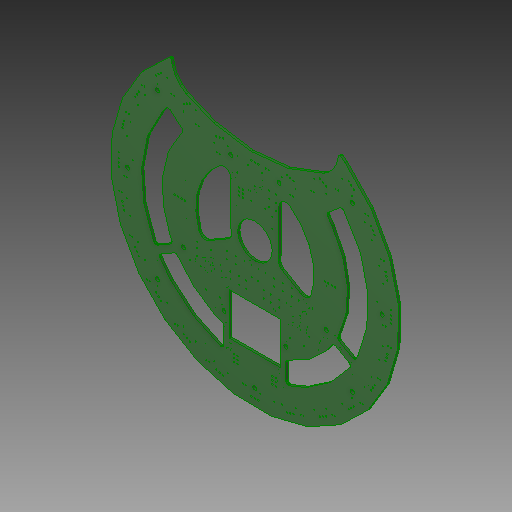
# Autodesk Inventor part: Board 2.brd_Outline
Saved by Autodesk Inventor 2017 (Build 210142000, 142)
## iProperties
Created: 2019-06-13
Part Number: Board 2.brd_Outline
Material: Generic
Document SubType Name: Modeling
Designer: Marc
Density: 1 g/cm^3
Appearance: Board Outline
Author: Marc
Autodesk Inventor part; units mm, degrees
ref_plane "YZ Plane" through (0, 0, 0) normal (1, 0, 0) x (0, 1, 0)
ref_plane "XZ Plane" through (0, 0, 0) normal (0, 1, 0) x (-1, 0, 0)
ref_plane "XY Plane" through (0, 0, 0) normal (0, 0, 1) x (1, 0, 0)
sketch "Sketch1" plane through (0, 0, 0) normal (0, 0, 1) x (1, 0, 0)
  line L0 (-60.7504, 83.7892) -> (-60.8105, 84.0432)
  line L1 (-60.8105, 84.0432) -> (-60.9343, 84.273)
  line L2 (-60.9343, 84.273) -> (-61.1134, 84.463)
  line L3 (-61.1134, 84.463) -> (-61.3355, 84.6001)
  line L4 (-61.3355, 84.6001) -> (-61.5856, 84.6751)
  line L5 (-61.5856, 84.6751) -> (-61.8465, 84.6827)
  line L6 (-61.8465, 84.6827) -> (-62.1005, 84.6226)
  line L7 (-62.1005, 84.6226) -> (-62.3304, 84.4988)
  line L8 (-62.3304, 84.4988) -> (-62.339, 84.4925)
  line L9 (-62.339, 84.4925) -> (-82.0829, 65.4791)
  line L10 (-82.0829, 65.4791) -> (-96.2331, 42.0034)
  line L11 (-96.2331, 42.0034) -> (-103.8251, 15.6653)
  line L12 (-103.8251, 15.6653) -> (-104.3417, -11.7403)
  line L13 (-104.3417, -11.7403) -> (-97.7475, -38.3458)
  line L14 (-97.7475, -38.3458) -> (-84.492, -62.338)
  line L15 (-84.492, -62.338) -> (-65.4786, -82.082)
  line L16 (-65.4786, -82.082) -> (-42.0029, -96.2321)
  line L17 (-42.0029, -96.2321) -> (-15.6648, -103.8242)
  line L18 (-15.6648, -103.8242) -> (11.7408, -104.3407)
  line L19 (11.7408, -104.3407) -> (38.3463, -97.7466)
  line L20 (38.3463, -97.7466) -> (62.3385, -84.4911)
  line L21 (62.3385, -84.4911) -> (82.0825, -65.4777)
  line L22 (82.0825, -65.4777) -> (96.2326, -42.002)
  line L23 (96.2326, -42.002) -> (103.8247, -15.6639)
  line L24 (103.8247, -15.6639) -> (104.3412, 11.7417)
  line L25 (104.3412, 11.7417) -> (97.7471, 38.3472)
  line L26 (97.7471, 38.3472) -> (84.4916, 62.3395)
  line L27 (84.4916, 62.3395) -> (65.4782, 82.0834)
  line L28 (65.4782, 82.0834) -> (62.338, 84.493)
  line L29 (62.338, 84.493) -> (62.1094, 84.6192)
  line L30 (62.1094, 84.6192) -> (61.8561, 84.682)
  line L31 (61.8561, 84.682) -> (61.5951, 84.6771)
  line L32 (61.5951, 84.6771) -> (61.3442, 84.6048)
  line L33 (61.3442, 84.6048) -> (61.1206, 84.47)
  line L34 (61.1206, 84.47) -> (60.9396, 84.282)
  line L35 (60.9396, 84.282) -> (60.8133, 84.0535)
  line L36 (60.8133, 84.0535) -> (60.7505, 83.8001)
  line L37 (60.7505, 83.8001) -> (60.7494, 83.7897)
  line L38 (60.7494, 83.7897) -> (59.5029, 78.5248)
  line L39 (59.5029, 78.5248) -> (56.9362, 73.7619)
  line L40 (56.9362, 73.7619) -> (53.2243, 69.8257)
  line L41 (53.2243, 69.8257) -> (50.001, 67.6671)
  line L42 (50.001, 67.6671) -> (24.4028, 57.8709)
  line L43 (24.4028, 57.8709) -> (-2.8586, 55.0339)
  line L44 (-2.8586, 55.0339) -> (-29.9254, 59.3492)
  line L45 (-29.9254, 59.3492) -> (-50.0022, 67.6648)
  line L46 (-50.0022, 67.6648) -> (-54.3828, 70.8409)
  line L47 (-54.3828, 70.8409) -> (-57.7921, 75.0425)
  line L48 (-57.7921, 75.0425) -> (-59.9977, 79.9833)
  line L49 (-59.9977, 79.9833) -> (-60.7504, 83.7892)
  line L50 (-68.3444, -42.3485) -> (-58.7823, -36.8278)
  line L51 (-58.7823, -36.8278) -> (-58.2999, -36.628)
  line L52 (-58.2999, -36.628) -> (-57.7823, -36.5598)
  line L53 (-57.7823, -36.5598) -> (-57.2646, -36.628)
  line L54 (-57.2646, -36.628) -> (-56.7822, -36.8278)
  line L55 (-56.7822, -36.8278) -> (-56.368, -37.1457)
  line L56 (-56.368, -37.1457) -> (-56.1187, -37.4496)
  line L57 (-56.1187, -37.4496) -> (-44.5118, -50.6997)
  line L58 (-44.5118, -50.6997) -> (-29.871, -60.4941)
  line L59 (-29.871, -60.4941) -> (-23.7915, -63.1334)
  line L60 (-23.7915, -63.1334) -> (-23.3311, -63.3797)
  line L61 (-23.3311, -63.3797) -> (-22.9502, -63.7368)
  line L62 (-22.9502, -63.7368) -> (-22.6747, -64.1803)
  line L63 (-22.6747, -64.1803) -> (-22.5234, -64.6799)
  line L64 (-22.5234, -64.6799) -> (-22.4968, -65.0049)
  line L65 (-22.4968, -65.0049) -> (-22.4968, -76.6705)
  line L66 (-22.4968, -76.6705) -> (-22.565, -77.1882)
  line L67 (-22.565, -77.1882) -> (-22.7648, -77.6705)
  line L68 (-22.7648, -77.6705) -> (-23.0826, -78.0848)
  line L69 (-23.0826, -78.0848) -> (-23.4968, -78.4026)
  line L70 (-23.4968, -78.4026) -> (-23.9792, -78.6024)
  line L71 (-23.9792, -78.6024) -> (-24.4968, -78.6705)
  line L72 (-24.4968, -78.6705) -> (-25.0145, -78.6024)
  line L73 (-25.0145, -78.6024) -> (-25.1056, -78.5756)
  line L74 (-25.1056, -78.5756) -> (-44.5884, -69.3987)
  line L75 (-44.5884, -69.3987) -> (-61.0322, -55.4919)
  line L76 (-61.0322, -55.4919) -> (-69.0178, -45.1758)
  line L77 (-69.0178, -45.1758) -> (-69.2443, -44.7054)
  line L78 (-69.2443, -44.7054) -> (-69.3413, -44.1924)
  line L79 (-69.3413, -44.1924) -> (-69.3022, -43.6718)
  line L80 (-69.3022, -43.6718) -> (-69.1298, -43.179)
  line L81 (-69.1298, -43.179) -> (-68.8356, -42.7477)
  line L82 (-68.8356, -42.7477) -> (-68.4398, -42.4072)
  line L83 (-68.4398, -42.4072) -> (-68.3444, -42.3485)
  line L84 (68.359, -42.3528) -> (68.7732, -42.6706)
  line L85 (68.7732, -42.6706) -> (69.0911, -43.0848)
  line L86 (69.0911, -43.0848) -> (69.2909, -43.5671)
  line L87 (69.2909, -43.5671) -> (69.359, -44.0848)
  line L88 (69.359, -44.0848) -> (69.2909, -44.6024)
  line L89 (69.2909, -44.6024) -> (69.0911, -45.0847)
  line L90 (69.0911, -45.0847) -> (69.0324, -45.1802)
  line L91 (69.0324, -45.1802) -> (54.9837, -61.508)
  line L92 (54.9837, -61.508) -> (37.1878, -73.6434)
  line L93 (37.1878, -73.6434) -> (25.1119, -78.5853)
  line L94 (25.1119, -78.5853) -> (24.598, -78.6779)
  line L95 (24.598, -78.6779) -> (24.0778, -78.6344)
  line L96 (24.0778, -78.6344) -> (23.5865, -78.4577)
  line L97 (23.5865, -78.4577) -> (23.1576, -78.1599)
  line L98 (23.1576, -78.1599) -> (22.8205, -77.7612)
  line L99 (22.8205, -77.7612) -> (22.5981, -77.2888)
  line L100 (22.5981, -77.2888) -> (22.5054, -76.775)
  line L101 (22.5054, -76.775) -> (22.5032, -76.6801)
  line L102 (22.5032, -76.6801) -> (22.5032, -65.005)
  line L103 (22.5032, -65.005) -> (22.5713, -64.4873)
  line L104 (22.5713, -64.4873) -> (22.7711, -64.005)
  line L105 (22.7711, -64.005) -> (23.089, -63.5907)
  line L106 (23.089, -63.5907) -> (23.5032, -63.2729)
  line L107 (23.5032, -63.2729) -> (23.7979, -63.1335)
  line L108 (23.7979, -63.1335) -> (39.3291, -54.8225)
  line L109 (39.3291, -54.8225) -> (52.18, -42.7749)
  line L110 (52.18, -42.7749) -> (56.1254, -37.4494)
  line L111 (56.1254, -37.4494) -> (56.4695, -37.0567)
  line L112 (56.4695, -37.0567) -> (56.9034, -36.7664)
  line L113 (56.9034, -36.7664) -> (57.3978, -36.5983)
  line L114 (57.3978, -36.5983) -> (57.9188, -36.5638)
  line L115 (57.9188, -36.5638) -> (58.4309, -36.6654)
  line L116 (58.4309, -36.6654) -> (58.789, -36.8276)
  line L117 (58.789, -36.8276) -> (68.359, -42.3528)
  line L118 (60.5006, -29.8823) -> (66.1735, -13.2065)
  line L119 (66.1735, -13.2065) -> (67.337, 4.3693)
  line L120 (67.337, 4.3693) -> (63.912, 21.6475)
  line L121 (63.912, 21.6475) -> (56.1317, 37.4504)
  line L122 (56.1317, 37.4504) -> (52.9183, 41.868)
  line L123 (52.9183, 41.868) -> (52.6505, 42.3163)
  line L124 (52.6505, 42.3163) -> (52.5079, 42.8185)
  line L125 (52.5079, 42.8185) -> (52.5002, 43.3406)
  line L126 (52.5002, 43.3406) -> (52.6278, 43.8468)
  line L127 (52.6278, 43.8468) -> (52.8821, 44.3028)
  line L128 (52.8821, 44.3028) -> (53.2012, 44.6411)
  line L129 (53.2012, 44.6411) -> (61.6386, 51.721)
  line L130 (61.6386, 51.721) -> (62.079, 52.0015)
  line L131 (62.079, 52.0015) -> (62.577, 52.1585)
  line L132 (62.577, 52.1585) -> (63.0986, 52.1812)
  line L133 (63.0986, 52.1812) -> (63.6083, 52.0682)
  line L134 (63.6083, 52.0682) -> (64.0714, 51.8271)
  line L135 (64.0714, 51.8271) -> (64.4564, 51.4743)
  line L136 (64.4564, 51.4743) -> (64.4878, 51.436)
  line L137 (64.4878, 51.436) -> (75.6044, 32.9894)
  line L138 (75.6044, 32.9894) -> (77.3033, 28.7844)
  line L139 (77.3033, 28.7844) -> (77.3951, 28.5737)
  line L140 (77.3951, 28.5737) -> (82.1527, 7.5695)
  line L141 (82.1527, 7.5695) -> (81.3119, -13.9503)
  line L142 (81.3119, -13.9503) -> (74.9301, -34.5192)
  line L143 (74.9301, -34.5192) -> (73.6407, -37.1903)
  line L144 (73.6407, -37.1903) -> (73.3465, -37.6216)
  line L145 (73.3465, -37.6216) -> (72.9507, -37.9621)
  line L146 (72.9507, -37.9621) -> (72.4802, -38.1885)
  line L147 (72.4802, -38.1885) -> (71.9672, -38.2855)
  line L148 (71.9672, -38.2855) -> (71.4465, -38.2463)
  line L149 (71.4465, -38.2463) -> (70.9537, -38.0738)
  line L150 (70.9537, -38.0738) -> (70.8555, -38.0206)
  line L151 (70.8555, -38.0206) -> (61.2938, -32.5001)
  line L152 (61.2938, -32.5001) -> (60.8795, -32.1823)
  line L153 (60.8795, -32.1823) -> (60.5617, -31.7681)
  line L154 (60.5617, -31.7681) -> (60.3619, -31.2858)
  line L155 (60.3619, -31.2858) -> (60.2937, -30.7681)
  line L156 (60.2937, -30.7681) -> (60.3619, -30.2505)
  line L157 (60.3619, -30.2505) -> (60.5006, -29.8823)
  line L158 (-17.2054, -3.1967) -> (-17.1364, -4.5002)
  line L159 (-17.1364, -4.5002) -> (-17.407, -5.7771)
  line L160 (-17.407, -5.7771) -> (-17.999, -6.9405)
  line L161 (-17.999, -6.9405) -> (-18.8719, -7.911)
  line L162 (-18.8719, -7.911) -> (-19.6211, -8.4408)
  line L163 (-19.6211, -8.4408) -> (-33.5098, -16.4596)
  line L164 (-33.5098, -16.4596) -> (-34.7157, -16.9591)
  line L165 (-34.7157, -16.9591) -> (-36.0099, -17.1294)
  line L166 (-36.0099, -17.1294) -> (-37.304, -16.959)
  line L167 (-37.304, -16.959) -> (-38.5099, -16.4595)
  line L168 (-38.5099, -16.4595) -> (-39.5454, -15.6649)
  line L169 (-39.5454, -15.6649) -> (-40.34, -14.6293)
  line L170 (-40.34, -14.6293) -> (-40.7482, -13.7257)
  line L171 (-40.7482, -13.7257) -> (-42.913, -2.7112)
  line L172 (-42.913, -2.7112) -> (-42.1534, 8.4883)
  line L173 (-42.1534, 8.4883) -> (-38.5209, 19.1096)
  line L174 (-38.5209, 19.1096) -> (-32.2632, 28.4289)
  line L175 (-32.2632, 28.4289) -> (-25.4611, 34.6541)
  line L176 (-25.4611, 34.6541) -> (-24.3174, 35.2832)
  line L177 (-24.3174, 35.2832) -> (-23.0499, 35.5948)
  line L178 (-23.0499, 35.5948) -> (-21.7449, 35.5677)
  line L179 (-21.7449, 35.5677) -> (-20.4914, 35.2037)
  line L180 (-20.4914, 35.2037) -> (-19.3747, 34.5278)
  line L181 (-19.3747, 34.5278) -> (-18.4711, 33.5858)
  line L182 (-18.4711, 33.5858) -> (-17.8421, 32.4421)
  line L183 (-17.8421, 32.4421) -> (-17.5305, 31.1746)
  line L184 (-17.5305, 31.1746) -> (-17.5002, 30.6251)
  line L185 (-17.5002, 30.6251) -> (-17.5003, 0.0028)
  line L186 (-17.5003, 0.0028) -> (-17.2054, -3.1967)
  line L187 (17.5017, 30.6288) -> (17.6721, 31.9229)
  line L188 (17.6721, 31.9229) -> (18.1716, 33.1288)
  line L189 (18.1716, 33.1288) -> (18.9662, 34.1644)
  line L190 (18.9662, 34.1644) -> (20.0018, 34.959)
  line L191 (20.0018, 34.959) -> (21.2077, 35.4584)
  line L192 (21.2077, 35.4584) -> (22.5018, 35.6288)
  line L193 (22.5018, 35.6288) -> (23.7959, 35.4584)
  line L194 (23.7959, 35.4584) -> (25.0018, 34.9589)
  line L195 (25.0018, 34.9589) -> (25.4619, 34.6584)
  line L196 (25.4619, 34.6584) -> (33.564, 26.8881)
  line L197 (33.564, 26.8881) -> (39.3789, 17.2857)
  line L198 (39.3789, 17.2857) -> (42.5104, 6.5054)
  line L199 (42.5104, 6.5054) -> (42.7451, -4.7181)
  line L200 (42.7451, -4.7181) -> (40.7535, -13.7294)
  line L201 (40.7535, -13.7294) -> (40.1788, -14.9014)
  line L202 (40.1788, -14.9014) -> (39.3204, -15.8846)
  line L203 (39.3204, -15.8846) -> (38.2368, -16.6122)
  line L204 (38.2368, -16.6122) -> (37.0018, -17.0345)
  line L205 (37.0018, -17.0345) -> (35.6995, -17.1228)
  line L206 (35.6995, -17.1228) -> (34.4188, -16.871)
  line L207 (34.4188, -16.871) -> (33.5153, -16.4629)
  line L208 (33.5153, -16.4629) -> (19.6223, -8.4417)
  line L209 (19.6223, -8.4417) -> (18.5867, -7.6472)
  line L210 (18.5867, -7.6472) -> (17.7921, -6.6117)
  line L211 (17.7921, -6.6117) -> (17.2926, -5.4058)
  line L212 (17.2926, -5.4058) -> (17.1222, -4.1118)
  line L213 (17.1222, -4.1118) -> (17.2066, -3.1972)
  line L214 (17.2066, -3.1972) -> (17.5017, 0.0027)
  line L215 (17.5017, 0.0027) -> (17.5017, 30.6288)
  line L216 (18.5032, -39.9326) -> (18.5032, -70.4326)
  line L217 (18.5032, -70.4326) -> (-18.4968, -70.4326)
  line L218 (-18.4968, -70.4326) -> (-18.4968, -39.9326)
  line L219 (-18.4968, -39.9326) -> (18.5032, -39.9326)
  line L220 (-52.9183, 41.868) -> (-61.9509, 26.7463)
  line L221 (-61.9509, 26.7463) -> (-63.0375, 24.0738)
  line L222 (-63.0375, 24.0738) -> (-63.0533, 24.0309)
  line L223 (-63.0533, 24.0309) -> (-67.1237, 6.8924)
  line L224 (-67.1237, 6.8924) -> (-66.6197, -10.7157)
  line L225 (-66.6197, -10.7157) -> (-61.5755, -27.5933)
  line L226 (-61.5755, -27.5933) -> (-60.4969, -29.8839)
  line L227 (-60.4969, -29.8839) -> (-60.3287, -30.3782)
  line L228 (-60.3287, -30.3782) -> (-60.2942, -30.8992)
  line L229 (-60.2942, -30.8992) -> (-60.3957, -31.4113)
  line L230 (-60.3957, -31.4113) -> (-60.6263, -31.8797)
  line L231 (-60.6263, -31.8797) -> (-60.9703, -32.2725)
  line L232 (-60.9703, -32.2725) -> (-61.29, -32.5018)
  line L233 (-61.29, -32.5018) -> (-70.8449, -38.0183)
  line L234 (-70.8449, -38.0183) -> (-71.3273, -38.2181)
  line L235 (-71.3273, -38.2181) -> (-71.8449, -38.2862)
  line L236 (-71.8449, -38.2862) -> (-72.3626, -38.218)
  line L237 (-72.3626, -38.218) -> (-72.8449, -38.0182)
  line L238 (-72.8449, -38.0182) -> (-73.2591, -37.7004)
  line L239 (-73.2591, -37.7004) -> (-73.577, -37.2861)
  line L240 (-73.577, -37.2861) -> (-73.6301, -37.1879)
  line L241 (-73.6301, -37.1879) -> (-80.7466, -16.861)
  line L242 (-80.7466, -16.861) -> (-82.3596, 4.6152)
  line L243 (-82.3596, 4.6152) -> (-78.3593, 25.7771)
  line L244 (-78.3593, 25.7771) -> (-77.3821, 28.5775)
  line L245 (-77.3821, 28.5775) -> (-77.3484, 28.6628)
  line L246 (-77.3484, 28.6628) -> (-67.2921, 47.7083)
  line L247 (-67.2921, 47.7083) -> (-64.4878, 51.436)
  line L248 (-64.4878, 51.436) -> (-64.1117, 51.7982)
  line L249 (-64.1117, 51.7982) -> (-63.6547, 52.0507)
  line L250 (-63.6547, 52.0507) -> (-63.1479, 52.1763)
  line L251 (-63.1479, 52.1763) -> (-62.6259, 52.1665)
  line L252 (-62.6259, 52.1665) -> (-62.1242, 52.0219)
  line L253 (-62.1242, 52.0219) -> (-61.677, 51.7523)
  line L254 (-61.677, 51.7523) -> (-61.6386, 51.721)
  line L255 (-61.6386, 51.721) -> (-53.2011, 44.6411)
  line L256 (-53.2011, 44.6411) -> (-52.8484, 44.2561)
  line L257 (-52.8484, 44.2561) -> (-52.6073, 43.793)
  line L258 (-52.6073, 43.793) -> (-52.4943, 43.2833)
  line L259 (-52.4943, 43.2833) -> (-52.5171, 42.7617)
  line L260 (-52.5171, 42.7617) -> (-52.6741, 42.2637)
  line L261 (-52.6741, 42.2637) -> (-52.9183, 41.868)
  line L262 (12.5, 0) -> (12.3931, 1.6316)
  line L263 (12.3931, 1.6316) -> (12.0741, 3.2352)
  line L264 (12.0741, 3.2352) -> (10.8253, 6.25)
  line L265 (10.8253, 6.25) -> (8.8388, 8.8388)
  line L266 (8.8388, 8.8388) -> (6.25, 10.8253)
  line L267 (6.25, 10.8253) -> (3.2352, 12.0741)
  line L268 (3.2352, 12.0741) -> (0, 12.5)
  line L269 (0, 12.5) -> (-3.2352, 12.0741)
  line L270 (-3.2352, 12.0741) -> (-6.25, 10.8253)
  line L271 (-6.25, 10.8253) -> (-8.8388, 8.8388)
  line L272 (-8.8388, 8.8388) -> (-10.8253, 6.25)
  line L273 (-10.8253, 6.25) -> (-12.0741, 3.2352)
  line L274 (-12.0741, 3.2352) -> (-12.5, 0)
  line L275 (-12.5, 0) -> (-12.0741, -3.2352)
  line L276 (-12.0741, -3.2352) -> (-10.8253, -6.25)
  line L277 (-10.8253, -6.25) -> (-8.8388, -8.8388)
  line L278 (-8.8388, -8.8388) -> (-6.25, -10.8253)
  line L279 (-6.25, -10.8253) -> (-3.2352, -12.0741)
  line L280 (-3.2352, -12.0741) -> (0, -12.5)
  line L281 (0, -12.5) -> (3.2352, -12.0741)
  line L282 (3.2352, -12.0741) -> (6.25, -10.8253)
  line L283 (6.25, -10.8253) -> (8.8388, -8.8388)
  line L284 (8.8388, -8.8388) -> (10.8253, -6.25)
  line L285 (10.8253, -6.25) -> (12.0741, -3.2352)
  line L286 (12.0741, -3.2352) -> (12.5, 0)
  circle A0 centre (-8.64, -93.98) radius 0.405
  circle A1 centre (-6.6, -93.98) radius 0.405
  circle A2 centre (33.27, -92.71) radius 0.405
  circle A3 centre (35.31, -92.71) radius 0.405
  circle A4 centre (56.13, -81.28) radius 0.405
  circle A5 centre (58.17, -81.28) radius 0.405
  circle A6 centre (78.49, -63.5) radius 0.405
  circle A7 centre (76.45, -63.5) radius 0.405
  circle A8 centre (91.19, -41.91) radius 0.405
  circle A9 centre (89.15, -41.91) radius 0.405
  circle A10 centre (98.81, -17.78) radius 0.405
  circle A11 centre (96.77, -17.78) radius 0.405
  circle A12 centre (92.96, -6.35) radius 0.405
  circle A13 centre (95, -6.35) radius 0.405
  circle A14 centre (93.73, 34.29) radius 0.405
  circle A15 centre (91.69, 34.29) radius 0.405
  circle A16 centre (82.3, 57.15) radius 0.405
  circle A17 centre (80.26, 57.15) radius 0.405
  circle A18 centre (58.67, 62.23) radius 0.405
  circle A19 centre (60.71, 62.23) radius 0.405
  circle A20 centre (40.89, 52.07) radius 0.405
  circle A21 centre (42.93, 52.07) radius 0.405
  circle A22 centre (25.65, 41.91) radius 0.405
  circle A23 centre (27.69, 41.91) radius 0.405
  circle A24 centre (7.87, 49.53) radius 0.405
  circle A25 centre (9.91, 49.53) radius 0.405
  circle A26 centre (-27.69, 41.91) radius 0.405
  circle A27 centre (-25.65, 41.91) radius 0.405
  circle A28 centre (-42.93, 52.07) radius 0.405
  circle A29 centre (-40.89, 52.07) radius 0.405
  circle A30 centre (-60.71, 62.23) radius 0.405
  circle A31 centre (-58.67, 62.23) radius 0.405
  circle A32 centre (-82.3, 57.15) radius 0.405
  circle A33 centre (-80.26, 57.15) radius 0.405
  circle A34 centre (-93.73, 34.29) radius 0.405
  circle A35 centre (-91.69, 34.29) radius 0.405
  circle A36 centre (-92.96, -6.35) radius 0.405
  circle A37 centre (-95, -6.35) radius 0.405
  circle A38 centre (-98.81, -17.78) radius 0.405
  circle A39 centre (-96.77, -17.78) radius 0.405
  circle A40 centre (-91.19, -41.91) radius 0.405
  circle A41 centre (-89.15, -41.91) radius 0.405
  circle A42 centre (-78.49, -63.5) radius 0.405
  circle A43 centre (-76.45, -63.5) radius 0.405
  circle A44 centre (-58.17, -81.28) radius 0.405
  circle A45 centre (-56.13, -81.28) radius 0.405
  circle A46 centre (-33.27, -92.71) radius 0.405
  circle A47 centre (-35.31, -92.71) radius 0.405
  circle A48 centre (6.35, -27.94) radius 0.405
  circle A49 centre (11.43, -27.94) radius 0.405
  circle A50 centre (6.35, -33.02) radius 0.405
  circle A51 centre (11.43, -33.02) radius 0.405
  circle A52 centre (7.62, -16.51) radius 0.405
  circle A53 centre (2.54, -16.51) radius 0.405
  circle A54 centre (-7.62, -16.51) radius 0.405
  circle A55 centre (-2.54, -16.51) radius 0.405
  circle A56 centre (-6.35, -33.02) radius 0.405
  circle A57 centre (-11.43, -33.02) radius 0.405
  circle A58 centre (-6.35, -27.94) radius 0.405
  circle A59 centre (-11.43, -27.94) radius 0.405
  circle A60 centre (26.67, -16.51) radius 0.405
  circle A61 centre (26.67, -21.59) radius 0.405
  circle A62 centre (15.24, 36.83) radius 0.405
  circle A63 centre (10.16, 36.83) radius 0.405
  circle A64 centre (-41.91, -25.4) radius 0.405
  circle A65 centre (-41.91, -30.48) radius 0.405
  circle A66 centre (20.32, -16.51) radius 0.405
  circle A67 centre (20.32, -21.59) radius 0.405
  circle A68 centre (13.97, -16.51) radius 0.405
  circle A69 centre (13.97, -21.59) radius 0.405
  circle A70 centre (15.24, 31.75) radius 0.405
  circle A71 centre (10.16, 31.75) radius 0.405
  circle A72 centre (15.24, 26.67) radius 0.405
  circle A73 centre (10.16, 26.67) radius 0.405
  circle A74 centre (-20.32, -21.59) radius 0.405
  circle A75 centre (-20.32, -16.51) radius 0.405
  circle A76 centre (-13.97, -21.59) radius 0.405
  circle A77 centre (-13.97, -16.51) radius 0.405
  circle A78 centre (46.99, -40.64) radius 0.405
  circle A79 centre (39.37, -40.64) radius 0.405
  circle A80 centre (12.7, 13.97) radius 0.405
  circle A81 centre (12.7, 21.59) radius 0.405
  circle A82 centre (-46.99, -35.56) radius 0.405
  circle A83 centre (-39.37, -35.56) radius 0.405
  circle A84 centre (50.8, 0) radius 0.51
  circle A85 centre (53.34, 0) radius 0.51
  circle A86 centre (55.88, 0) radius 0.51
  circle A87 centre (58.42, 0) radius 0.51
  circle A88 centre (12.7, -78.74) radius 0.51
  circle A89 centre (15.24, -78.74) radius 0.51
  circle A90 centre (12.7, -81.28) radius 0.51
  circle A91 centre (15.24, -81.28) radius 0.51
  circle A92 centre (12.7, -83.82) radius 0.51
  circle A93 centre (15.24, -83.82) radius 0.51
  circle A94 centre (-11.43, 27.94) radius 0.51
  circle A95 centre (-8.89, 27.94) radius 0.51
  circle A96 centre (-11.43, 25.4) radius 0.51
  circle A97 centre (-8.89, 25.4) radius 0.51
  circle A98 centre (-11.43, 22.86) radius 0.51
  circle A99 centre (-8.89, 22.86) radius 0.51
  circle A100 centre (-58.42, 0) radius 0.51
  circle A101 centre (-55.88, 0) radius 0.51
  circle A102 centre (-53.34, 0) radius 0.51
  circle A103 centre (-50.8, 0) radius 0.51
  circle A104 centre (-12.7, -83.82) radius 0.51
  circle A105 centre (-15.24, -83.82) radius 0.51
  circle A106 centre (-12.7, -81.28) radius 0.51
  circle A107 centre (-15.24, -81.28) radius 0.51
  circle A108 centre (-12.7, -78.74) radius 0.51
  circle A109 centre (-15.24, -78.74) radius 0.51
  circle A110 centre (17.78, -28.07) radius 0.405
  circle A111 centre (17.78, -32.89) radius 0.405
  circle A112 centre (2.41, -24.13) radius 0.405
  circle A113 centre (-2.41, -24.13) radius 0.405
  circle A114 centre (-17.78, -32.89) radius 0.405
  circle A115 centre (-17.78, -28.07) radius 0.405
  circle A116 centre (13.97, -94.23) radius 0.405
  circle A117 centre (3.81, -94.23) radius 0.405
  circle A118 centre (19.68, -93.08) radius 0.405
  circle A119 centre (29.49, -90.45) radius 0.405
  circle A120 centre (43.1, -84.81) radius 0.405
  circle A121 centre (51.9, -79.73) radius 0.405
  circle A122 centre (63.58, -70.77) radius 0.405
  circle A123 centre (70.77, -63.58) radius 0.405
  circle A124 centre (79.73, -51.9) radius 0.405
  circle A125 centre (84.81, -43.1) radius 0.405
  circle A126 centre (90.45, -29.49) radius 0.405
  circle A127 centre (93.08, -19.68) radius 0.405
  circle A128 centre (99.06, 6.1) radius 0.405
  circle A129 centre (88.9, 6.1) radius 0.405
  circle A130 centre (93.08, 19.68) radius 0.405
  circle A131 centre (90.45, 29.49) radius 0.405
  circle A132 centre (84.81, 43.1) radius 0.405
  circle A133 centre (79.73, 51.9) radius 0.405
  circle A134 centre (70.77, 63.58) radius 0.405
  circle A135 centre (63.58, 70.77) radius 0.405
  circle A136 centre (51.9, 55.6) radius 0.405
  circle A137 centre (43.1, 60.68) radius 0.405
  circle A138 centre (29.49, 47.27) radius 0.405
  circle A139 centre (19.68, 49.9) radius 0.405
  circle A140 centre (5.08, 45.47) radius 0.405
  circle A141 centre (-5.08, 45.47) radius 0.405
  circle A142 centre (-19.68, 49.9) radius 0.405
  circle A143 centre (-29.49, 47.27) radius 0.405
  circle A144 centre (-43.1, 60.68) radius 0.405
  circle A145 centre (-51.9, 55.6) radius 0.405
  circle A146 centre (-63.58, 70.77) radius 0.405
  circle A147 centre (-70.77, 63.58) radius 0.405
  circle A148 centre (-79.73, 51.9) radius 0.405
  circle A149 centre (-84.81, 43.1) radius 0.405
  circle A150 centre (-90.45, 29.49) radius 0.405
  circle A151 centre (-93.08, 19.68) radius 0.405
  circle A152 centre (-99.06, 6.6) radius 0.405
  circle A153 centre (-88.9, 6.6) radius 0.405
  circle A154 centre (-93.08, -19.68) radius 0.405
  circle A155 centre (-90.45, -29.49) radius 0.405
  circle A156 centre (-84.81, -43.1) radius 0.405
  circle A157 centre (-79.73, -51.9) radius 0.405
  circle A158 centre (-70.77, -63.58) radius 0.405
  circle A159 centre (-63.58, -70.77) radius 0.405
  circle A160 centre (-51.9, -79.73) radius 0.405
  circle A161 centre (-43.1, -84.81) radius 0.405
  circle A162 centre (-29.49, -90.45) radius 0.405
  circle A163 centre (-19.68, -93.08) radius 0.405
  circle A164 centre (35.81, -48.26) radius 0.405
  circle A165 centre (25.65, -48.26) radius 0.405
  circle A166 centre (7.62, 24.13) radius 0.405
  circle A167 centre (-2.54, 24.13) radius 0.405
  circle A168 centre (-35.56, -48.26) radius 0.405
  circle A169 centre (-25.4, -48.26) radius 0.405
  circle A170 centre (41.91, -21.59) radius 0.405
  circle A171 centre (31.75, -21.59) radius 0.405
  circle A172 centre (-12.7, 46.99) radius 0.405
  circle A173 centre (-12.7, 36.83) radius 0.405
  circle A174 centre (-41.91, -21.59) radius 0.405
  circle A175 centre (-31.75, -21.59) radius 0.405
  circle A176 centre (0, -99.01) radius 0.525
  circle A177 centre (2.54, -99.01) radius 0.525
  circle A178 centre (-2.54, -99.01) radius 0.525
  circle A179 centre (25.63, -95.64) radius 0.525
  circle A180 centre (28.08, -94.98) radius 0.525
  circle A181 centre (23.17, -96.29) radius 0.525
  circle A182 centre (49.51, -85.75) radius 0.525
  circle A183 centre (51.7, -84.48) radius 0.525
  circle A184 centre (47.31, -87.02) radius 0.525
  circle A185 centre (70.01, -70.01) radius 0.525
  circle A186 centre (71.81, -68.21) radius 0.525
  circle A187 centre (68.21, -71.81) radius 0.525
  circle A188 centre (85.75, -49.51) radius 0.525
  circle A189 centre (87.02, -47.31) radius 0.525
  circle A190 centre (84.48, -51.7) radius 0.525
  circle A191 centre (95.64, -25.63) radius 0.525
  circle A192 centre (96.29, -23.17) radius 0.525
  circle A193 centre (94.98, -28.08) radius 0.525
  circle A194 centre (99.01, 0) radius 0.525
  circle A195 centre (99.01, 2.54) radius 0.525
  circle A196 centre (99.01, -2.54) radius 0.525
  circle A197 centre (95.64, 25.63) radius 0.525
  circle A198 centre (94.98, 28.08) radius 0.525
  circle A199 centre (96.29, 23.17) radius 0.525
  circle A200 centre (85.75, 49.51) radius 0.525
  circle A201 centre (84.48, 51.7) radius 0.525
  circle A202 centre (87.02, 47.31) radius 0.525
  circle A203 centre (70.01, 70.01) radius 0.525
  circle A204 centre (68.21, 71.81) radius 0.525
  circle A205 centre (71.81, 68.21) radius 0.525
  circle A206 centre (49.51, 61.62) radius 0.525
  circle A207 centre (47.31, 62.89) radius 0.525
  circle A208 centre (51.7, 60.35) radius 0.525
  circle A209 centre (25.63, 52.46) radius 0.525
  circle A210 centre (23.17, 53.11) radius 0.525
  circle A211 centre (28.08, 51.8) radius 0.525
  circle A212 centre (0, 49.48) radius 0.525
  circle A213 centre (-2.54, 49.48) radius 0.525
  circle A214 centre (2.54, 49.48) radius 0.525
  circle A215 centre (-25.63, 52.46) radius 0.525
  circle A216 centre (-28.08, 51.8) radius 0.525
  circle A217 centre (-23.17, 53.11) radius 0.525
  circle A218 centre (-49.51, 61.62) radius 0.525
  circle A219 centre (-51.7, 60.35) radius 0.525
  circle A220 centre (-47.31, 62.89) radius 0.525
  circle A221 centre (-70.01, 70.01) radius 0.525
  circle A222 centre (-71.81, 68.21) radius 0.525
  circle A223 centre (-68.21, 71.81) radius 0.525
  circle A224 centre (-85.75, 49.51) radius 0.525
  circle A225 centre (-87.02, 47.31) radius 0.525
  circle A226 centre (-84.48, 51.7) radius 0.525
  circle A227 centre (-95.64, 25.63) radius 0.525
  circle A228 centre (-96.29, 23.17) radius 0.525
  circle A229 centre (-94.98, 28.08) radius 0.525
  circle A230 centre (-99.01, 0) radius 0.525
  circle A231 centre (-99.01, -2.54) radius 0.525
  circle A232 centre (-99.01, 2.54) radius 0.525
  circle A233 centre (-95.64, -25.63) radius 0.525
  circle A234 centre (-94.98, -28.08) radius 0.525
  circle A235 centre (-96.29, -23.17) radius 0.525
  circle A236 centre (-85.75, -49.51) radius 0.525
  circle A237 centre (-84.48, -51.7) radius 0.525
  circle A238 centre (-87.02, -47.31) radius 0.525
  circle A239 centre (-70.01, -70.01) radius 0.525
  circle A240 centre (-68.21, -71.81) radius 0.525
  circle A241 centre (-71.81, -68.21) radius 0.525
  circle A242 centre (-49.51, -85.75) radius 0.525
  circle A243 centre (-47.31, -87.02) radius 0.525
  circle A244 centre (-51.7, -84.48) radius 0.525
  circle A245 centre (-25.63, -95.64) radius 0.525
  circle A246 centre (-23.17, -96.29) radius 0.525
  circle A247 centre (-28.08, -94.98) radius 0.525
  circle A248 centre (-70.8591, 59.4579) radius 1.5
  circle A249 centre (-92.4893, 0) radius 1.5
  circle A250 centre (-70.8591, -59.4579) radius 1.5
  circle A251 centre (0, -92.5) radius 1.5
  circle A252 centre (-22.4968, -55.1826) radius 1.5
  circle A253 centre (22.4968, -55.1826) radius 1.5
  circle A254 centre (70.8591, -59.4579) radius 1.5
  circle A255 centre (51.8178, -29.9159) radius 1.5
  circle A256 centre (92.4893, 0) radius 1.5
  circle A257 centre (70.8591, 59.4579) radius 1.5
  circle A258 centre (17.5002, 45.5508) radius 1.5
  circle A259 centre (-17.5002, 45.5508) radius 1.5
  circle A260 centre (-51.8178, -29.9159) radius 1.5
  circle A261 centre (-30.7086, -29.0322) radius 0.3048
  circle A262 centre (32.9946, -30.5562) radius 0.3048
  circle A263 centre (33.2232, -39.3954) radius 0.3048
  circle A264 centre (27.7368, -33.6042) radius 0.175
  circle A265 centre (27.7368, -37.4904) radius 0.175
  circle A266 centre (46.4058, -45.4914) radius 0.175
  circle A267 centre (61.9506, -36.195) radius 0.175
  circle A268 centre (70.485, -41.4528) radius 0.175
  circle A269 centre (16.2306, -79.9338) radius 0.175
  circle A270 centre (-20.955, -33.6042) radius 0.175
  circle A271 centre (-21.1074, -62.103) radius 0.175
  circle A272 centre (-18.5928, -73.0758) radius 0.175
  circle A273 centre (34.4424, -27.813) radius 0.175
  circle A274 centre (37.4904, -37.1094) radius 0.175
  circle A275 centre (52.6542, -35.1282) radius 0.175
  circle A276 centre (63.0174, -36.8046) radius 0.175
  circle A277 centre (70.7898, -48.387) radius 0.175
  circle A278 centre (-24.4602, -31.0134) radius 0.175
  circle A279 centre (-31.9278, -26.289) radius 0.175
  circle A280 centre (32.385, -37.1856) radius 0.175
  circle A281 centre (31.242, -39.0906) radius 0.175
  circle A282 centre (27.5844, -39.4716) radius 0.175
  circle A283 centre (15.1638, -36.576) radius 0.175
  circle A284 centre (26.289, -28.1178) radius 0.175
  circle A285 centre (24.6888, -40.5384) radius 0.175
  circle A286 centre (17.3736, -72.39) radius 0.175
  circle A287 centre (-24.765, -27.5082) radius 0.175
  circle A288 centre (-30.3276, -30.5562) radius 0.175
  circle A289 centre (-37.6428, -29.1846) radius 0.175
  circle A290 centre (-14.0208, 33.0708) radius 0.175
  circle A291 centre (-50.3682, 13.0302) radius 0.175
  circle A292 centre (35.6616, -19.2786) radius 0.175
  circle A293 centre (-0.3048, 32.385) radius 0.175
  circle A294 centre (33.2994, -32.2326) radius 0.175
  circle A295 centre (37.4142, -27.2796) radius 0.175
  circle A296 centre (37.4142, -20.4978) radius 0.175
  circle A297 centre (-34.7472, -36.957) radius 0.175
  circle A298 centre (-36.1188, -36.576) radius 0.175
  circle A299 centre (-16.3068, 35.1282) radius 0.175
  circle A300 centre (5.0292, 34.8996) radius 0.175
  circle A301 centre (-29.8704, -26.2128) radius 0.175
  circle A302 centre (-43.2054, -32.9184) radius 0.175
  circle A303 centre (-70.485, -47.7774) radius 0.175
  circle A304 centre (-35.6616, -82.6008) radius 0.175
  circle A305 centre (22.7076, -51.6636) radius 0.175
  circle A306 centre (18.1356, -74.4474) radius 0.175
  circle A307 centre (20.955, -81.8388) radius 0.175
  circle A308 centre (13.6398, -35.9664) radius 0.175
  circle A309 centre (-20.3454, -39.243) radius 0.175
  circle A310 centre (32.8422, -34.5948) radius 0.175
  circle A311 centre (37.4142, -39.1668) radius 0.175
  circle A312 centre (47.7774, -39.1668) radius 0.175
  circle A313 centre (51.8922, -2.3622) radius 0.175
  circle A314 centre (49.8348, -35.7378) radius 0.175
  circle A315 centre (36.3474, -26.289) radius 0.175
  circle A316 centre (39.9288, -22.2504) radius 0.175
  circle A317 centre (5.4102, 37.1094) radius 0.175
  circle A318 centre (5.4102, 40.8432) radius 0.175
  circle A319 centre (3.6576, 35.5092) radius 0.175
  circle A320 centre (-49.911, -10.8966) radius 0.175
  circle A321 centre (-36.4236, -28.575) radius 0.175
  circle A322 centre (-33.3756, -29.7942) radius 0.175
  circle A323 centre (-43.053, -34.5948) radius 0.175
  circle A324 centre (-35.9664, -30.48) radius 0.175
  circle A325 centre (-36.7284, -34.8996) radius 0.175
  circle A326 centre (-32.3088, -31.3182) radius 0.175
  circle A327 centre (-19.3548, -38.1) radius 0.175
  circle A328 centre (-19.6596, -76.7334) radius 0.175
  circle A329 centre (-20.6502, -77.724) radius 0.175
  circle A330 centre (-17.0688, -76.0476) radius 0.175
  circle A331 centre (-28.8036, -56.2356) radius 0.175
  circle A332 centre (34.8234, -26.8986) radius 0.175
  circle A333 centre (39.243, -22.86) radius 0.175
  circle A334 centre (58.293, -30.2514) radius 0.175
  circle A335 centre (82.3722, -49.6062) radius 0.175
  circle A336 centre (1.3716, 31.3944) radius 0.175
  circle A337 centre (-23.8506, -34.8234) radius 0.175
  circle A338 centre (-23.8506, -51.9684) radius 0.175
  circle A339 centre (-20.4978, -61.4172) radius 0.175
  circle A340 centre (-17.3736, -73.3806) radius 0.175
  circle A341 centre (-17.6784, -77.5716) radius 0.175
  circle A342 centre (22.9362, -27.2796) radius 0.3048
  circle A343 centre (38.3286, -34.8996) radius 0.3048
  circle A344 centre (-0.1524, 34.4424) radius 0.3048
  circle A345 centre (-31.4706, -34.4424) radius 0.3048
  circle A346 centre (-29.337, -32.1564) radius 0.3048
  circle A347 centre (-4.7244, 29.7942) radius 0.175
  circle A348 centre (-13.6398, 15.6972) radius 0.175
  circle A349 centre (-3.3528, 29.7942) radius 0.175
  circle A350 centre (-3.6576, -14.0208) radius 0.175
  constraints: 574 end point, 351 centre point
extrude "Board 2.brd_Outline" add sketch "Sketch1" along normal blind 1.6
body "Solid1"
